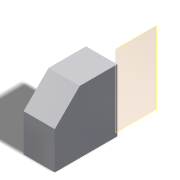
# Autodesk Inventor part: 00_STORMModule
Saved by Autodesk Inventor 2019.4 (Build 234330000, 330)
## iProperties
Created: 2020-10-09
Part Number: 00_STORMModule
Material: Generic
Document SubType Name: Modeling
Designer: diederichbenedict
Density: 1 g/cm^3
Appearance: White
Author: diederichbenedict
Autodesk Inventor part; units mm, degrees
ref_plane "YZ Plane" through (0, 0, 0) normal (1, 0, 0) x (0, 1, 0)
ref_plane "XZ Plane" through (0, 0, 0) normal (0, 1, 0) x (-1, 0, 0)
ref_plane "XY Plane" through (0, 0, 0) normal (0, 0, 1) x (1, 0, 0)
ref_plane "Work Plane1" through (225, -51.9999, -200.9642) normal (1, 0, 0) x (0, 0, -1)
sketch "Sketch1" plane through (225, -51.9999, -200.9642) normal (1, 0, 0) x (0, 0, -1)
  line L0 (-200.9642, 89.4999) -> (-130.9642, 89.4999) projected
  line L1 (-130.9642, 89.4999) -> (-130.9642, 14.4999) projected
  line L2 (-130.9642, 14.4999) -> (-200.9642, 14.4999) projected
  line L3 (-200.9642, 14.4999) -> (-200.9642, -53.5599) projected
  line L4 (-200.9642, -53.5599) -> (-122.2497, -53.5599) projected
  ellipse E0 centre (-122.3295, -48.5209) end of major axis (-118.6887, -52.0634) minor radius 5 (-122.2497, -53.5599) -> (-117.3008, -48.2463) ccw projected
  line L5 (-117.3008, -48.2463) -> (-117.6163, -43.7662) projected
  line L6 (-117.6163, -43.7662) -> (-94.1545, -42.114) projected
  line L7 (-94.1545, -42.114) -> (-81.3155, 140.1971) projected
  arc A0 (-81.3155, 140.1971) -> (-85.9519, 145.536) centre (-86.3031, 140.5484) ccw projected
  line L8 (-85.9519, 145.536) -> (-117.6163, 147.7659) projected
  line L9 (-117.6163, 147.7659) -> (-117.3008, 152.246) projected
  ellipse E1 centre (-122.3295, 152.5206) end of major axis (-118.6887, 156.0631) minor radius 5 (-117.3008, 152.246) -> (-122.2497, 157.5596) ccw projected
  line L10 (-122.2497, 157.5596) -> (-200.9642, 157.5596) projected
  line L11 (-200.9642, 89.4999) -> (-200.9642, 157.5596) projected
  line L12 (-200.9642, 123.5297) -> (-400.9642, 123.5297)
  line L13 (-400.9642, 123.5297) -> (-400.9642, -76.4703)
  line L14 (-400.9642, -76.4703) -> (-200.9642, -76.4703)
  line L15 (-200.9642, -76.4703) -> (-200.9642, 123.5297)
  line L16 (-348.854, 122.9439) -> (-400.9642, 70.8337)
  line L17 (-347.4398, 123.5297) -> (-273.7448, 123.5297) construction
  arc A1 (-347.4398, 123.5297) -> (-348.854, 122.9439) centre (-347.4398, 121.5297) ccw
  point P0 (-200.9642, 51.9999)
  point P1 (-348.2682, 123.5297)
  dimension "d0" = 200
  dimension "d1" = 200
  dimension "d2" = 135
  dimension "d3" = 2
  constraints: 12 end point, 4 point on line, 2 horizontal, 2 parallel, 2 point on circle, 2 tangent, 1 centre point, 1 equal length, 1 midpoint, 1 perpendicular, 2 other
  measures "d0" distance of L14.end L13.end
  measures "d1" distance of L13.end L12.end
  measures "d2" angle of L16 L17
  measures "d3" radius of A1
extrude "Extrusion1" add sketch "Sketch1" against normal blind 100 contours L15 L3 L14 L13 L16 A1 L12 L11 | A1 L16 L13 L12
chamfer "Chamfer1" distance 80 angle 45 1 edges at (175, 71.5299, 200)
body "Solid1"
